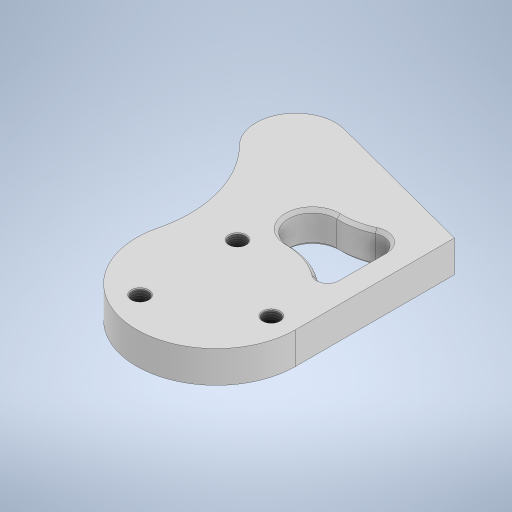
# Autodesk Inventor part: Curve
Saved by Autodesk Inventor 2023.2 (Build 272271000, 271)
## iProperties
Created: 2023-01-17
Part Number: Curve
Material: Generic
Document SubType Name: Modeling
Designer: manas
Density: 1 g/cm^3
Appearance: Default
Author: manas
Autodesk Inventor part; units mm, degrees
ref_plane "YZ Plane" through (0, 0, 0) normal (1, 0, 0) x (0, 1, 0)
ref_plane "XZ Plane" through (0, 0, 0) normal (0, 1, 0) x (-1, 0, 0)
ref_plane "XY Plane" through (0, 0, 0) normal (0, 0, 1) x (1, 0, 0)
sketch "Sketch1" plane through (0, 0, 0) normal (0, 1, 0) x (-1, 0, 0)
  line L0 (0, 0) -> (0, -100)
  arc A0 (93.6713, -124.5596) -> (117.8498, -82.8611) centre (100.0117, -100.377) ccw
  line L1 (0, -100) -> (93.6713, -124.5596)
  arc A1 (98.5447, -12.3594) -> (0, 0) centre (49.9985, -0.39) ccw
  arc A2 (99.0048, -10.5865) -> (117.8498, -82.8611) centre (171.3639, -30.3137) ccw
  arc A3 (49.1416, -75.3835) -> (49.6184, -45.3884) centre (49.5087, -60.388) ccw
  arc A4 (22.9948, -36.4248) -> (49.6184, -45.3884) centre (49.9477, -0.3896) ccw
  line L2 (15, -40.4287) -> (15, -70.4287)
  arc A5 (22.9948, -36.4248) -> (15, -40.4287) centre (20, -40.4287) ccw
  arc A6 (15, -70.4287) -> (29.3397, -79.438) centre (25, -70.4287) ccw
  arc A7 (49.1416, -75.3835) -> (29.1892, -79.5089) centre (48.0406, -120.37) ccw
  circle A8 centre (14.9985, 0) radius 5
  circle A9 centre (67.085, -30.8513) radius 5
  circle A10 centre (67.7598, 29.6826) radius 5
  dimension "d0" = 100
  dimension "d3" = 50
  dimension "d5" = 50
  dimension "d6" = 75
  dimension "d13" = 15
  dimension "d14" = 60
  dimension "d16" = 45
  dimension "d17" = 5
  dimension "d19" = 10
  dimension "d24" = 30
  dimension "d25" = 15
  dimension "d26" = 45
  dimension "d57" = 10
  dimension "d58" = 35
  dimension "d61" = 360
  constraints: 18 point on circle, 11 centre point, 9 tangent, 6 end point, 2 vertical, 7 other
  measures "d0" distance of L0.start L0.end
  measures "d3" diameter of A0
  measures "d5" radius of A1
  measures "d6" radius of A2
  measures "d13" radius of A3
  measures "d14" distance of A1.centre A3.centre
  measures "d16" radius of A4
  measures "d17" radius of A5
  measures "d19" radius of A6
  measures "d24" vertical distance of A6.centre A5.centre
  measures "d25" distance between parallel lines of L2 L0
  measures "d26" radius of A7
  measures "d57" diameter of A8
  measures "d58" horizontal distance of A1.centre A8.centre
extrude "Extrusion2" add sketch "Sketch1" along normal blind 20
chamfer "Chamfer2" distance 2 angle 45 12 edges at (-64.5068, 20, -60.6264) (-38.9289, 20, -76.3021) (-19.6098, 20, -78.8516) (-15, 20, -55.4287) (-17.761, 20, -35.958) (-35.5892, 20, -43.0373) (-64.5068, 0, -60.6264) (-38.9289, 0, -76.3021) (-19.6098, 0, -78.8516) (-15, 0, -55.4287) (-17.761, 0, -35.958) (-35.5892, 0, -43.0373)
chamfer "Chamfer3" distance 0.5 angle 45 3 edges at (-62.085, 20, -30.8513) (-62.7598, 20, 29.6826) (-9.9985, 20, 0)
thread "Thread1" size "M10x1.25" class "6H" standard "ANSI Metric M Profile" full length
thread "Thread2" size "M10x1.5" class "6H" standard "ANSI Metric M Profile" full length
thread "Thread3" size "M10x1.5" class "6H" standard "ANSI Metric M Profile" full length
body "Solid2"
